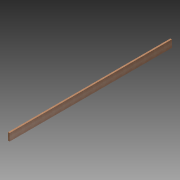
# Autodesk Inventor part: Support Board
Saved by Autodesk Inventor 2015 (Build 190159000, 159)
## iProperties
Created: 2014-05-27
Part Number: Support Board
Material: Wood (Birch)
Document SubType Name: Modeling
Designer: Haden
Density: 0.55 g/cm^3
Appearance: Birch - Natural Polished
Mass: 15682.4 g
Surface Area: 18204.8 cm^2
Volume: 28513.5 cm^3
Author: Haden
Autodesk Inventor part; units mm, degrees
ref_plane "YZ Plane" through (0, 0, 0) normal (1, 0, 0) x (0, 1, 0)
ref_plane "XZ Plane" through (0, 0, 0) normal (0, 1, 0) x (-1, 0, 0)
ref_plane "XY Plane" through (0, 0, 0) normal (0, 0, 1) x (1, 0, 0)
sketch "Sketch1" plane through (0, 0, 0) normal (0, 0, 1) x (1, 0, 0)
  line L0 (0, 0) -> (38.1, 0)
  line L1 (38.1, 0) -> (38.1, -184.15)
  line L2 (38.1, -184.15) -> (0, -184.15)
  line L3 (0, -184.15) -> (0, 0)
  dimension "d0" = 38.1
  dimension "d1" = 184.15
  constraints: 8 end point, 2 parallel, 1 horizontal, 1 perpendicular
  measures "d0" distance of L1.end L2.end
  measures "d1" distance of L0.end L1.end
extrude "Extrusion1" add sketch "Sketch1" along normal blind 4064
body "Solid1"
